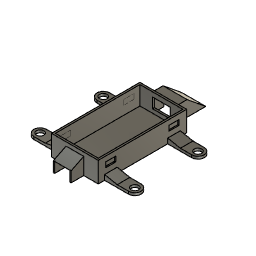
cage_protection_controlleur_moteur v12 (Autodesk Fusion 360 design; units mm, degrees)
Autodesk Fusion 360 part; units mm, degrees
sketch "Esquisse1" plane through (0, 0, 0) normal (0, 0, 1) x (1, 0, 0)
  line L0 (-9, 50) -> (25, 50)
  line L1 (25, 50) -> (25, -17)
  line L2 (25, -17) -> (-9, -17)
  line L3 (-9, -17) -> (-9, 50)
  line L4 (-10.5, 51.5) -> (26.5, 51.5)
  line L5 (26.5, 51.5) -> (26.5, -18.5)
  line L6 (26.5, -18.5) -> (-10.5, -18.5)
  line L7 (-10.5, -18.5) -> (-10.5, 51.5)
  circle A0 centre (45.5, -8.5) radius 3
  circle A1 centre (-29.5, -8.5) radius 3
  circle A2 centre (-29.5, 41.5) radius 3
  circle A3 centre (45.5, 41.5) radius 3
  line L8 (26.5, -13.5) -> (26.5, -3.5)
  line L9 (26.5, -13.5) -> (45.5, -13.5)
  line L10 (26.5, -3.5) -> (45.5, -3.5)
  arc A4 (45.5, -13.5) -> (45.5, -3.5) centre (45.5, -8.5) ccw
  line L11 (8, 51.5) -> (8, -18.5) construction
  line L12 (-10.5, 16.5) -> (26.5, 16.5) construction
  line L13 (-10.5, -3.5) -> (-29.5, -3.5)
  line L14 (-10.5, -13.5) -> (-29.5, -13.5)
  arc A5 (-29.5, -3.5) -> (-29.5, -13.5) centre (-29.5, -8.5) ccw
  line L15 (-10.5, 36.5) -> (-29.5, 36.5)
  arc A6 (-29.5, 46.5) -> (-29.5, 36.5) centre (-29.5, 41.5) ccw
  line L16 (-10.5, 46.5) -> (-29.5, 46.5)
  line L17 (26.5, 36.5) -> (45.5, 36.5)
  arc A7 (45.5, 36.5) -> (45.5, 46.5) centre (45.5, 41.5) ccw
  line L18 (26.5, 46.5) -> (45.5, 46.5)
  dimension "d1" = 34
  dimension "d2" = 67
  dimension "d3" = 70
  dimension "d4" = 37
  dimension "d5" = 1.5
  dimension "d6" = 1.5
  dimension "d32" = 50
  dimension "d33" = 50
  dimension "d34" = 75
  dimension "d35" = 6
  dimension "d36" = 6
  dimension "d37" = 6
  dimension "d38" = 6
  dimension "d46" = 10
  dimension "d73" = 25
  dimension "d74" = 75
  dimension "d76" = 25
  dimension "d77" = 37.5
  dimension "d79" = 37.5
  dimension "d80" = 37.5
  dimension "d81" = 25
  constraint horizontal L0
  constraint vertical L1
  constraint horizontal L2
  constraint vertical L3
  constraint horizontal L4
  constraint vertical L5
  constraint horizontal L6
  constraint vertical L7
  constraint vertical L8
  constraint coincident L5 L8.end
  constraint perpendicular L8 L9
  constraint perpendicular L8 L10
  constraint tangent L9 A4
  constraint midpoint L4 L11.start
  constraint midpoint L6 L11.end
  constraint midpoint L7 L12.start
  constraint midpoint L5 L12.end
  constraint symmetric L8.start L11 L14.start
  constraint symmetric L8.end L11 L13.start
  constraint symmetric L9.end L11 L14.end
  constraint symmetric L10.end L11 L13.end
  constraint symmetric A4 L11 A5
  constraint symmetric L8.start L12 L18.start
  constraint symmetric L8.end L12 L17.start
  constraint symmetric L9.end L12 A7.end
  constraint symmetric L10.end L12 L17.end
  constraint symmetric A4 L12 A7
  constraint symmetric L12 L13.start L15.start
  constraint symmetric L12 L13.end L15.end
  constraint symmetric L12 L14.start L16.start
  constraint symmetric L12 L14.end A6.start
  constraint symmetric L12 A5 A6
  measures "d1" distance of L1 L3
  measures "d2" distance of L0 L2
  measures "d3" distance of L4 L6
  measures "d4" distance of L5 L7
  measures "d5" distance of L1 L5
  measures "d6" distance of L0 L4
  measures "d32" distance of A0.centre A3.centre
  measures "d33" distance of A1.centre A2.centre
  measures "d34" distance of A0.centre A1.centre
  measures "d35" diameter of A0
  measures "d36" diameter of A3
  measures "d37" diameter of A1
  measures "d38" diameter of A2
  measures "d46" distance of L9 L10
  measures "d73" distance of A3.centre L12
  measures "d74" distance of A2.centre A3.centre
  measures "d76" distance of A2.centre L12
  measures "d77" distance of A2.centre L11
  measures "d79" distance of L9.end L11
  measures "d80" distance of L10.end L11
  measures "d81" distance of A0.centre L12
extrude "Extrusion1" add sketch "Esquisse1" along normal blind 1.5 contours L0 L1 L2 L3
extrude "Extrusion2" add sketch "Esquisse1" along normal blind 14.2 contours L4 L5 L6 L7 L8
sketch "Esquisse3" plane through (0, -18.5, 0) normal (0, -1, 0) x (1, 0, 0)
  line L0 (-10.5, 0) -> (26.5, 0)
  line L1 (26.5, 0) -> (26.5, 14.2)
  line L2 (26.5, 14.2) -> (-10.5, 14.2)
  line L3 (-10.5, 14.2) -> (-10.5, 0)
  line L4 (-7.1003, 3.1205) -> (-7.1003, 1.5002)
  line L5 (5, 5.9405) -> (11, 5.9405)
  line L6 (-7.1003, 1.5002) -> (24.8997, 1.5002)
  line L7 (24.8997, 3.1205) -> (-7.1003, 3.1205)
  line L8 (3.9, 4.5655) -> (3.9, 4.7655)
  line L9 (12.1, 4.7655) -> (12.1, 4.5655)
  line L10 (24.8997, 3.1205) -> (24.8997, 1.5002)
  line L11 (5, 2.7405) -> (11, 2.7405)
  line L12 (8, 5.9405) -> (8, 2.7405) construction
  line L13 (2.1378, 4.3405) -> (15.1, 4.3405) construction
  arc A0 (5, 5.9405) -> (3.9, 4.7655) centre (5.0776, 4.7655) ccw
  arc A1 (3.9, 4.5655) -> (5, 2.7405) centre (5.9639, 4.5655) ccw
  arc A2 (12.1, 4.7655) -> (11, 5.9405) centre (10.9224, 4.7655) ccw
  arc A3 (11, 2.7405) -> (12.1, 4.5655) centre (9.84, 4.6837) ccw
  point P0 (-7.1003, 3.1205)
  point P1 (-7.1003, 3.1205)
  dimension "d61" = 18.5
  dimension "d66" = 4.1
  dimension "d67" = 4.1
  dimension "d68" = 6
  dimension "d69" = 1.6
  dimension "d70" = 1.6
  dimension "d71" = 4.3405
  constraint parallel L7 L11
  constraint perpendicular L11 L12
  constraint midpoint L5 L12.start
  constraint midpoint L11 L12.end
  constraint horizontal L13
  constraint tangent L8 A0
  constraint tangent L8 A1
  constraint tangent L9 A2
  constraint tangent A2 A3
  measures "d61" distance of L3 L12
  measures "d66" distance of L9 L12
  measures "d67" distance of L8 L12
  measures "d68" distance of L11.start L11.end
  measures "d69" distance of L5 L13
  measures "d70" distance of L11 L13
  measures "d71" distance of L0 L13
extrude "Extrusion3" cut sketch "Esquisse3" against normal up to surface (1.5 mm away) contours L5 L7 L8 L9 A0 A1 A2 A3 | L7 L11 A1 A3
extrude "Extrusion4" add 1 faces at (-10, 27.6667, 14.2) along direction (0, 0, 1) blind 1
sketch "Esquisse4" plane through (0, 0, 15.2) normal (0, 0, 1) x (-1, 0, 0)
  line L0 (9.5, 4.5) -> (9.5, 12.5)
  line L1 (10.5, 12.5) -> (10.5, 4.5)
  line L2 (10.5, 4.5) -> (9.5, 4.5)
  line L3 (9.5, 12.5) -> (10.5, 12.5)
  line L4 (10.5, 18.5) -> (-26.5, 18.5) construction
  line L5 (-8, 18.5) -> (-8, -51.5) construction
  line L6 (10.5, -51.5) -> (-26.5, -51.5)
  line L7 (-8, -16.5) -> (10.5, -16.5) construction
  line L8 (10.5, 18.5) -> (10.5, -51.5)
  line L9 (9.5, -45.5) -> (10.5, -45.5)
  line L10 (9.5, -37.5) -> (9.5, -45.5)
  line L11 (10.5, -45.5) -> (10.5, -37.5)
  line L12 (10.5, -37.5) -> (9.5, -37.5)
  line L13 (-26.5, -37.5) -> (-25.5, -37.5)
  line L14 (-25.5, -37.5) -> (-25.5, -45.5)
  line L15 (-26.5, -45.5) -> (-26.5, -37.5)
  line L16 (-25.5, -45.5) -> (-26.5, -45.5)
  line L17 (-25.5, 4.5) -> (-25.5, 12.5)
  line L18 (-26.5, 12.5) -> (-26.5, 4.5)
  line L19 (-25.5, 12.5) -> (-26.5, 12.5)
  line L20 (-26.5, 4.5) -> (-25.5, 4.5)
  point P0 (10.5, 13.5)
  point P1 (10.5, 18.5)
  point P2 (-26.5, 18.5)
  dimension "d82" = 8
  dimension "d83" = 1
  dimension "d84" = 21
  constraint coincident L1 P0
  constraint coincident L4 P1
  constraint coincident P1 L4.start
  constraint coincident P2 L4.end
  constraint midpoint L4 L5.start
  constraint perpendicular L4 L5
  constraint coincident L5.end L6
  constraint midpoint L5 L7.start
  constraint perpendicular L5 L7
  constraint coincident L7.end L8
  constraint symmetric L1.start L7 L9.end
  constraint symmetric L0.end L7 L9.start
  constraint symmetric L1.end L7 L11.end
  constraint symmetric L0.start L7 L10.start
  constraint symmetric L1.start L5 L18.start
  constraint symmetric L0.end L5 L17.end
  constraint symmetric L1.end L5 L18.end
  constraint symmetric L0.start L5 L17.start
  constraint symmetric L5 L9.start L14.end
  constraint symmetric L5 L9.end L15.start
  constraint symmetric L5 L10.start L13.end
  constraint symmetric L5 L11.end L13.start
  measures "d82" distance of L2 L3
  measures "d83" distance of L0 L1
  measures "d84" distance of L2 L7
extrude "Extrusion5" cut sketch "Esquisse4" against normal blind 4 from surface at -3
extrude "Extrusion6" add sketch "Esquisse1" along normal blind 2 contours L7 L15 A6 L16 | L5 L17 A7 L18 | L7 L13 L14 A5 | L5 L8 L9 L10 A4
sketch "Esquisse5" plane through (0, -13.5, 0) normal (0, -1, 0) x (1, 0, 0)
  line L0 (26.5, 0) -> (45.5, 0)
  line L1 (45.5, 0) -> (45.5, 2)
  line L2 (45.5, 2) -> (26.5, 2)
  line L3 (26.5, 2) -> (26.5, 0)
  line L4 (26.5, 2) -> (26.5, 4)
  line L5 (26.5, 4) -> (36.5, 2)
  line L6 (8, 1) -> (8, 17.4128) construction
  line L7 (-10.5, 4) -> (-20.5, 2)
  line L8 (-10.5, 2) -> (-10.5, 4)
  line L9 (-20.5, 2) -> (-10.5, 2)
  dimension "d50" = 2
  dimension "d51" = 10
  dimension "d52" = 18.5
  constraint coincident L2 L3.start
  constraint perpendicular L2 L4
  constraint coincident L2.end L4
  constraint vertical L6
  constraint symmetric L2.end L6 L8.start
  constraint symmetric L4.end L6 L7.start
  constraint symmetric L5.end L6 L7.end
  constraint perpendicular L8 L9
  measures "d50" distance of L2.end L4.end
  measures "d51" distance of L2.end L5.end
  measures "d52" distance of L4 L6
sketch "Esquisse6" plane through (0, 46.5, 0) normal (0, 1, 0) x (-1, 0, 0)
  line L0 (-45.5, 0) -> (-26.5, 0)
  line L1 (-26.5, 0) -> (-26.5, 2)
  line L2 (-26.5, 2) -> (-45.5, 2)
  line L3 (-45.5, 2) -> (-45.5, 0)
  line L4 (10.5, 2) -> (10.5, 0)
  line L5 (10.5, 2) -> (10.5, 4)
  line L6 (10.5, 4) -> (20.5, 2)
  line L7 (-26.5, 4) -> (-36.5, 2)
  line L8 (-8, 1) -> (-8, 17.4128) construction
  line L9 (-26.5, 2) -> (-26.5, 4)
  line L10 (-36.5, 2) -> (-26.5, 2)
  line L11 (10.5, 2) -> (20.5, 2)
  point P0 (1.5244, 2.1172)
  point P1 (10.5, 2)
  dimension "d53" = 2
  dimension "d54" = 10
  dimension "d56" = 18.5
  dimension "d72" = 18.5
  constraint coincident P1 L5
  constraint vertical L8
  constraint symmetric L1.end P1 L8
  constraint symmetric L7.start L5.end L8
  constraint symmetric L6.end L7.end L8
  constraint coincident L4.end L5
  constraint perpendicular L9 L10
  constraint perpendicular L4 L11
  constraint coincident L11 P1
  measures "d53" distance of L5.end P1
  measures "d54" distance of L6.end P1
  measures "d56" distance of L1.end L8
  measures "d72" distance of L5 L8
extrude "Extrusion7" add sketch "Esquisse5" against normal up to surface (10 mm away) contours L2 L4 L5 | L7 L8 L9
extrude "Extrusion8" add sketch "Esquisse6" against normal up to surface (10 mm away) contours L2 L7 L9 L10 | L5 L6 L11
sketch "Esquisse7" plane through (0, 51.5, 0) normal (0, 1, 0) x (-1, 0, 0)
  line L0 (-26.5, 0) -> (10.5, 0)
  line L1 (10.5, 0) -> (10.5, 15.2)
  line L2 (10.5, 15.2) -> (-26.5, 15.2)
  line L3 (-26.5, 15.2) -> (-26.5, 0)
  line L4 (-15, 12.6) -> (-1, 12.6)
  line L5 (-1, 12.6) -> (-1, 4.6)
  line L6 (-1, 4.6) -> (-15, 4.6)
  line L7 (-15, 4.6) -> (-15, 12.6)
  line L8 (-8, 15.2) -> (-8, 0) construction
  line L9 (-26.5, 7.6) -> (10.5, 7.6) construction
  dimension "d85" = 8
  dimension "d86" = 14
  dimension "d87" = 7
  dimension "d88" = 5
  constraint horizontal L4
  constraint vertical L5
  constraint horizontal L6
  constraint vertical L7
  constraint midpoint L2 L8.start
  constraint midpoint L0 L8.end
  constraint midpoint L3 L9.start
  constraint midpoint L1 L9.end
  measures "d85" distance of L4 L6
  measures "d86" distance of L5 L7
  measures "d87" distance of L7 L8
  measures "d88" distance of L4 L9
extrude "Extrusion9" cut sketch "Esquisse7" against normal up to surface (1.5 mm away) contours L4 L5 L6 L7
extrude "Extrusion10" add 1 faces at (-10, 27.6667, 15.2) along direction (0, 0, 1) blind 1
sketch "Esquisse8" plane through (26.5, 0, 0) normal (1, 0, 0) x (0, 1, 0)
  line L0 (46.5, 4) -> (46.5, 0)
  line L1 (46.5, 0) -> (51.5, 0)
  line L2 (51.5, 0) -> (51.5, 16.2)
  line L3 (51.5, 16.2) -> (-18.5, 16.2)
  line L4 (-18.5, 16.2) -> (-18.5, 0)
  line L5 (-18.5, 0) -> (-13.5, 0)
  line L6 (-13.5, 0) -> (-13.5, 4)
  line L7 (-13.5, 4) -> (-3.5, 4)
  line L8 (-3.5, 4) -> (-3.5, 0)
  line L9 (-3.5, 0) -> (36.5, 0)
  line L10 (36.5, 0) -> (36.5, 4)
  line L11 (36.5, 4) -> (46.5, 4)
  line L12 (45.5, 12.2) -> (45.5, 8.2)
  line L13 (45.5, 8.2) -> (37.5, 8.2)
  line L14 (37.5, 8.2) -> (37.5, 12.2)
  line L15 (37.5, 12.2) -> (45.5, 12.2)
  line L16 (-4.5, 12.2) -> (-4.5, 8.2)
  line L17 (-4.5, 8.2) -> (-12.5, 8.2)
  line L18 (-12.5, 8.2) -> (-12.5, 12.2)
  line L19 (-12.5, 12.2) -> (-4.5, 12.2)
  line L20 (-18.5, 13.2) -> (-28.5, 8.2)
  line L21 (-28.5, 8.2) -> (-18.5, 8.2)
  line L22 (-18.5, 12.082) -> (-26.2639, 8.2)
  line L23 (-28.5, 8.2) -> (-18.5, 8.2)
  line L24 (-18.5, 8.2) -> (-18.5, 0)
  line L25 (-18.5, 0) -> (-28.5, 0)
  line L26 (-28.5, 0) -> (-28.5, 8.2)
  line L27 (60.5, 12.7) -> (60.5, 0)
  line L28 (60.5, 0) -> (51.5, 0)
  line L29 (51.5, 0) -> (51.5, 12.7)
  line L30 (51.5, 12.7) -> (51.5, 13.7)
  line L31 (51.5, 13.7) -> (60.8568, 13.7)
  line L32 (51.5, 12.7) -> (60.5, 12.7)
  line L33 (76.1148, 1.6) -> (60.5, 1.6)
  line L34 (60.8568, 13.7) -> (75.6542, 1.6)
  line L35 (60.5, 12.7) -> (74.0745, 1.6)
  point P0 (51.5, 4.6)
  dimension "d93" = 1
  dimension "d95" = 3
  dimension "d98" = 5
  dimension "d100" = 10
  dimension "d106" = 9
  dimension "d116" = 1
  dimension "d118" = 9
  dimension "d119" = 2.5
  dimension "d120" = 3
  dimension "d132" = 1
  constraint coincident L4 L20.start
  constraint perpendicular L4 L21
  constraint coincident L4 L22.start
  constraint parallel L20 L22
  constraint coincident L4 L21.end
  constraint horizontal L23
  constraint vertical L24
  constraint horizontal L25
  constraint vertical L26
  constraint coincident L4.end L5.start
  constraint coincident L2 L29.end
  constraint vertical L27
  constraint horizontal L28
  constraint vertical L29
  constraint coincident L1.end L28
  constraint coincident L2 L30.end
  constraint perpendicular L30 L31
  constraint perpendicular L30 L32
  constraint coincident L27.start L32
  constraint coincident L27 L33.end
  constraint perpendicular L27 L33
  constraint parallel L34 L35
  constraint coincident L33 L34.end
  constraint coincident L33 L35.end
  constraint coincident L22.end L23
  measures "d93" distance of L20 L22
  measures "d95" distance of L3.end L20.start
  measures "d98" distance of L20.start L21
  measures "d100" distance of L20.end L21.end
  measures "d106" distance of L27 L29
  measures "d116" distance of L29.end L30.end
  measures "d118" distance of L29.end L27.start
  measures "d119" distance of L3 L31
  measures "d120" distance of L33 P0
  measures "d132" distance of L34 L35
extrude "Extrusion12" add sketch "Esquisse8" against normal blind 1 from surface at -11.5 contours L4 L20 L21 L22 L23 | L4 L21 L23 L24 L25 L26 | L4 L21 L22 L23
extrude "Extrusion13" add sketch "Esquisse8" against normal blind 12 from surface at -12.5 contours L4 L20 L21 L22 L23
extrude "Extrusion14" add 1 faces at (15, -21.8333, 7.1333) along direction (-1, 0, 0) blind 1 from surface at 13
extrude "Extrusion15" add sketch "Esquisse8" along normal blind 1 from surface at -10 contours L2 L27 L28 L29 L32 | L2 L30 L31 L32 L33 L34 L35 | L27 L33 L35
extrude "Extrusion16" add sketch "Esquisse8" against normal blind 17 from surface at -10 contours L2 L30 L31 L32 L33 L34 L35
extrude "Extrusion17" add sketch "Esquisse8" against normal blind 1 from surface at -27 contours L2 L27 L28 L29 L32 | L2 L30 L31 L32 L33 L34 L35 | L27 L33 L35
equation "d9 = 1.5 mm + 12.7 mm"
